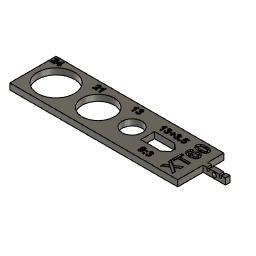
Test_Board (Autodesk Fusion 360 design; units mm, degrees)
Autodesk Fusion 360 part; units mm, degrees
note: some values were not read from the file. Set by a fixed rule: which sketch regions a step uses.
sketch "Esboço1" plane through (0, 0, 0) normal (0, 0, 1) x (1, 0, 0)
  circle A0 centre (0, 0) radius 12
  circle A1 centre (27.5, -0.1039) radius 10.5
  circle A2 centre (49.5, -0.1039) radius 6.5
  line L0 (72.3807, 4.6105) -> (75.8807, 1.6105)
  line L1 (59.3807, 4.6105) -> (59.3807, -4.3895)
  line L2 (59.3807, -4.3895) -> (72.3807, -4.3895)
  line L3 (72.3807, -4.3895) -> (75.8807, -1.3895)
  line L4 (75.8807, 1.6105) -> (75.8807, -1.3895)
  line L5 (59.3807, 4.6105) -> (72.3807, 4.6105)
  line L6 (0, 0) -> (-15, 0)
  line L7 (-15, 0) -> (-15, 15)
  line L8 (-15, 15) -> (0, 15)
  line L9 (0, 15) -> (0, 0)
  line L10 (-15, 15) -> (108.5, 15)
  line L11 (108.5, 15) -> (108.5, -15)
  line L12 (108.5, -15) -> (-15, -15)
  line L13 (-15, -15) -> (-15, 15)
  line L14 (-13.8356, 11.1144) -> (-8.721, 11.0985) construction
  line L15 (-8.721, 11.0985) -> (-8.7144, 13.2394) construction
  line L16 (-8.7144, 13.2394) -> (-13.8289, 13.2553) construction
  line L17 (-13.8289, 13.2553) -> (-13.8356, 11.1144) construction
  line L18 (14.4394, 9.9375) -> (19.5539, 9.9216) construction
  line L19 (19.5539, 9.9216) -> (19.5606, 12.0625) construction
  line L20 (19.5606, 12.0625) -> (14.4461, 12.0784) construction
  line L21 (14.4461, 12.0784) -> (14.4394, 9.9375) construction
  line L22 (39.4394, 9.9375) -> (44.5539, 9.9216) construction
  line L23 (44.5539, 9.9216) -> (44.5606, 12.0625) construction
  line L24 (44.5606, 12.0625) -> (39.4461, 12.0784) construction
  line L25 (39.4461, 12.0784) -> (39.4394, 9.9375) construction
  line L26 (61.7177, 8.0773) -> (73.2699, 8.0463) construction
  line L27 (73.2699, 8.0463) -> (73.2765, 10.5209) construction
  line L28 (73.2765, 10.5209) -> (61.7244, 10.5519) construction
  line L29 (61.7244, 10.5519) -> (61.7177, 8.0773) construction
  line L30 (62.0513, -10.4606) -> (73.6035, -10.4916) construction
  line L31 (73.6035, -10.4916) -> (73.6092, -8.3505) construction
  line L32 (73.6092, -8.3505) -> (62.0571, -8.3195) construction
  line L33 (62.0571, -8.3195) -> (62.0513, -10.4606) construction
  line L34 (85.7189, -5.7319) -> (85.7499, 5.8203) construction
  line L35 (85.7499, 5.8203) -> (83.6089, 5.826) construction
  line L36 (83.6089, 5.826) -> (83.5779, -5.7261) construction
  line L37 (83.5779, -5.7261) -> (85.7189, -5.7319) construction
  line L38 (72.3807, 4.6105) -> (72.3807, -4.3895)
  line L39 (94, -15) -> (108.5, -15)
  line L40 (108.5, -15) -> (108.5, 1.5)
  line L41 (108.5, 1.5) -> (94, 1.5)
  line L42 (94, 1.5) -> (94, -15)
  line L43 (108.5, 1.5) -> (94, 1.5)
  line L44 (94, 1.5) -> (94, 4.5)
  line L45 (94, 4.5) -> (108.5, 4.5)
  line L46 (108.5, 4.5) -> (108.5, 1.5)
  line L47 (94, 4.5) -> (94, 15)
  line L48 (56.5044, 15) -> (56.5044, -15)
  line L49 (79.6258, 15) -> (79.6258, -15)
  dimension "d1" = 24
  dimension "d2" = 21
  dimension "d3" = 13
  dimension "d4" = 27.5
  dimension "d5" = 22
  dimension "d7" = 15
  dimension "d8" = 15
  dimension "d9" = 123.5
  dimension "d10" = 30
  dimension "d13" = 4
  dimension "d14" = 4
  dimension "d15" = 4
  dimension "d16" = 4
  dimension "d17" = 4
  dimension "d21" = 8
  dimension "d22" = 9
  dimension "d23" = 3
  dimension "d24" = 13
  dimension "d25" = 3.5
  dimension "d29" = 16.5
  dimension "d30" = 14.5
  dimension "d31" = 3
  dimension "d32" = 109
  text T0 "24" font "Arial" height 4 bold align centre middle in box 5.1146 x 2.1409 at (-13.8356, 11.1144) x (0.999995, -0.003112) y (0.003112, 0.999995) spacing 1
  text T1 "21" font "Arial" height 4 bold align centre middle in box 5.1146 x 2.1409 at (14.4394, 9.9375) x (0.999995, -0.003112) y (0.003112, 0.999995) spacing 1
  text T2 "13" font "Arial" height 4 bold align centre middle in box 5.1146 x 2.1409 at (39.4394, 9.9375) x (0.999995, -0.003112) y (0.003112, 0.999995) spacing 1
  text T3 "13+3.5" font "Arial" height 4 bold align centre middle in box 11.5522 x 2.4746 at (61.7177, 8.0773) x (0.999996, -0.002682) y (0.002682, 0.999996) spacing 1
  text T4 "9:3" font "Arial" height 4 bold align centre middle in box 11.5522 x 2.141 at (62.0513, -10.4606) x (0.999996, -0.002682) y (0.002682, 0.999996) spacing 1
  text T5 "XT60" font "Arial" height 8 bold align centre middle in box 11.5522 x 2.141 at (85.7189, -5.7319) x (0.002682, 0.999996) y (-0.999996, 0.002682) spacing 1
  constraint coincident A0.centre L6.start
  constraint vertical L1
  constraint perpendicular L1 L2
  constraint parallel L1 L4
  constraint perpendicular L1 L5
  constraint horizontal L6
  constraint vertical L7
  constraint horizontal L8
  constraint vertical L9
  constraint horizontal L10
  constraint vertical L11
  constraint horizontal L12
  constraint vertical L13
  constraint equal L2 L5
  constraint equal L0 L3
  constraint horizontal L39
  constraint vertical L40
  constraint horizontal L41
  constraint vertical L42
  constraint coincident L12 L39.start
  constraint horizontal L43
  constraint vertical L44
  constraint horizontal L45
  constraint vertical L46
  constraint equal L41 L45
  constraint coincident L10 L47.end
  constraint perpendicular L10 L47
  constraint coincident L10 L48.start
  constraint coincident L12 L48.end
  constraint perpendicular L12 L48
  constraint coincident L10 L49.start
  constraint coincident L12 L49.end
  constraint perpendicular L12 L49
  measures "d1" diameter of A0
  measures "d2" diameter of A1
  measures "d3" diameter of A2
  measures "d4" horizontal distance of A0.centre A1.centre
  measures "d5" distance of A1.centre A2.centre
  measures "d7" distance of A0.centre L6.end
  measures "d8" distance of A0.centre L8.end
  measures "d9" distance of L7.end L10.end
  measures "d10" distance of L7.end L12.end
  measures "d22" distance of L1.start L1.end
  measures "d23" distance of L0.end L3.end
  measures "d24" distance of L1.start L0.start
  measures "d25" distance of L4 L38
  measures "d29" distance of L39 L41
  measures "d30" distance of L40.end L41.end
  measures "d31" distance of L40.end L45.end
  measures "d32" distance of L12.end L39.start
extrude "Extrusão1" add sketch "Esboço1" along normal blind 4 contours A0 L6 L9 L10 L12 L13 L48 | A0 L6 L7 L8 L9 L10 L13 | L10 L12 L48 L49 | L10 L12 L42 L44 L47 L49 | L11 L41 L43 L44 L45 L46
extrude "Extrusão2" cut sketch "Esboço1" against normal blind 1 from surface at 4 text T0 T1 T2 T3 T4 T5
sketch "Esboço2" plane through (0, 1.5, 0) normal (0, -1, 0) x (1, 0, 0)
  line L0 (94, 0) -> (108.5, 0)
  line L1 (108.5, 0) -> (108.5, 4)
  line L2 (108.5, 4) -> (94, 4)
  line L3 (94, 4) -> (94, 0)
  line L4 (101.25, 4) -> (101.25, 0)
  circle A0 centre (101.25, 2) radius 1.4
  line L5 (94, 2) -> (108.5, 2)
  line L6 (94, 2.8) -> (108.5, 2.8)
  circle A1 centre (97.25, 2.8) radius 0.75
  circle A2 centre (105.25, 2.8) radius 0.75
  line L7 (96.5, 2) -> (96.5, 4)
  line L8 (106, 4) -> (106, 2)
  line L9 (98, 2) -> (98, 4)
  line L10 (104.5, 4) -> (104.5, 2)
  dimension "d33" = 2.8
  dimension "d36" = 0.8
  dimension "d37" = 1.5
  dimension "d38" = 1.5
  dimension "d39" = 4
  dimension "d40" = 4
  constraint midpoint L2 L4.start
  constraint midpoint L0 L4.end
  constraint midpoint L4 A0.centre
  constraint midpoint L3 L5.start
  constraint midpoint L1 L5.end
  constraint coincident L3 L6.start
  constraint coincident L1 L6.end
  constraint perpendicular L1 L6
  constraint coincident L6 A1.centre
  constraint coincident L6 A2.centre
  constraint coincident L5 L7.start
  constraint coincident L2 L7.end
  constraint perpendicular L2 L7
  constraint tangent A1 L7
  constraint coincident L2 L8.start
  constraint coincident L5 L8.end
  constraint perpendicular L5 L8
  constraint tangent A2 L8
  constraint coincident L5 L9.start
  constraint coincident L2 L9.end
  constraint perpendicular L2 L9
  constraint tangent A1 L9
  constraint coincident L2 L10.start
  constraint coincident L5 L10.end
  constraint perpendicular L5 L10
  constraint tangent A2 L10
  measures "d33" diameter of A0
  measures "d36" distance of L5 L6
  measures "d37" diameter of A1
  measures "d38" diameter of A2
  measures "d39" distance of L4 A1.centre
  measures "d40" distance of L4 A2.centre
extrude "Extrusão3" cut sketch "Esboço2" against normal blind 3 contours L4 A0 L5 | L4 A0 L5 | L4 A0 L5 L6 | L4 A0 L5 L6 | L6 A1 | L2 A1 L7 L9 | L6 A1 | L4 A0 L6 | L4 A0 L6 | L6 A2 | L6 A2 | L2 A2 L8 L10
equation "d4 = d1 / 2 + d2 / 2 + 5 mm"
equation "d5 = d2 / 2 + d3 / 2 + 5 mm"
equation "d7 = d1 / 2 + 3 mm"
equation "d8 = d1 / 2 + 3 mm"
equation "d9 = d32 + d30"
equation "d10 = d1 + 6 mm"
